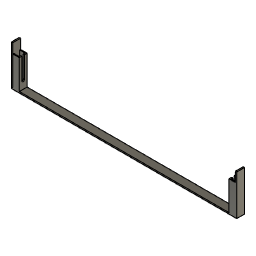
motor_base1 v1 (Autodesk Fusion 360 design; units mm, degrees)
Autodesk Fusion 360 part; units mm, degrees
sketch "Sketch1" plane through (0, 0, 0) normal (0, 0, 1) x (1, 0, 0)
  line L0 (-173, 6) -> (173, 6)
  line L1 (173, 6) -> (173, -6)
  line L2 (173, -6) -> (-173, -6)
  line L3 (-173, -6) -> (-173, 6)
  dimension "d1" = 346
  dimension "d2" = 12
  constraint horizontal L0
  constraint perpendicular L0 L1
  constraint parallel L0 L2
  constraint parallel L1 L3
  measures "d1" distance of L0.start L0.end
  measures "d2" distance of L0.end L1.end
extrude "Extrude1" add sketch "Sketch1" along normal blind 2
sketch "Sketch2" plane through (0, 0, 2) normal (0, 0, 1) x (-1, 0, 0)
  line L0 (173, 6) -> (-173, 6)
  line L1 (-173, 6) -> (-173, -6)
  line L2 (-173, -6) -> (173, -6)
  line L3 (173, -6) -> (173, 6)
  line L4 (-171, 6) -> (-171, -6)
  line L5 (-171, 6) -> (-173, 6)
  line L6 (-173, -6) -> (-171, -6)
  line L7 (171, 6) -> (171, -6)
  line L8 (171, 6) -> (173, 6)
  line L9 (173, -6) -> (171, -6)
  dimension "d9" = 2
  dimension "d10" = 2
  constraint coincident L0 L4.start
  constraint perpendicular L0 L4
  constraint coincident L0.end L1.start
  constraint coincident L1.end L2.start
  constraint coincident L0 L7.start
  constraint coincident L2 L7.end
  constraint perpendicular L2 L7
  constraint coincident L0.start L3.end
  constraint coincident L2.end L3.start
  measures "d9" distance of L1 L4
  measures "d10" distance of L3 L7
extrude "Extrude2" add sketch "Sketch2" along normal blind 60 contours L0 L2 L3 L7 L8 L9 | L0 L1 L2 L4 L5 L6
sketch "Sketch3" plane through (171, 0, 0) normal (-1, 0, 0) x (0, -1, 0)
  line L0 (-6, 2) -> (6, 2)
  line L1 (6, 2) -> (6, 62)
  line L2 (6, 62) -> (-6, 62)
  line L3 (-6, 62) -> (-6, 2)
  line L4 (-6, 62) -> (-6, 47)
  line L5 (-6, 47) -> (6, 47)
  line L6 (6, 47) -> (6, 0)
  line L7 (6, 0) -> (-6, 0)
  line L8 (-6, 0) -> (-6, 47)
  dimension "d13" = 15
  constraint coincident L2.end L3.start
  constraint perpendicular L2 L4
  constraint coincident L1 L5.end
  constraint perpendicular L1 L5
  constraint perpendicular L0 L6
  constraint perpendicular L3 L7
  constraint perpendicular L5 L8
  measures "d13" distance of L2.end L4.end
extrude "Extrude3" add sketch "Sketch3" along normal blind 10 contours L0 L1 L3 L5 L6 L8
sketch "Sketch4" plane through (0, 0, 47) normal (0, 0, 1) x (-1, 0, 0)
  line L0 (-171, 6) -> (-171, -6)
  line L1 (-171, -6) -> (-161, -6)
  line L2 (-161, -6) -> (-161, 6)
  line L3 (-161, 6) -> (-171, 6)
  line L4 (-171, 4.5) -> (-170, 4.5)
  line L5 (-170, 4.5) -> (-163, 4.5)
  line L6 (-163, 4.5) -> (-163, -4.5)
  line L7 (-163, -4.5) -> (-171, -4.5)
  line L8 (-171, 4.5) -> (-171, 3.6158)
  dimension "d16" = 1.5
  dimension "d17" = 1.5
  dimension "d18" = 8
  constraint coincident L0 L4.start
  constraint perpendicular L0 L4
  constraint perpendicular L0 L5
  constraint perpendicular L4 L6
  constraint coincident L0 L7.end
  constraint perpendicular L0 L7
  constraint coincident L0 L8.end
  measures "d16" distance of L3 L5
  measures "d17" distance of L1 L7
  measures "d18" distance of L6.end L7.end
extrude "Extrude4" cut sketch "Sketch4" against normal blind 43 contours L0 L4 L5 L6 L7 L8
sketch "Sketch5" plane through (161, 0, 0) normal (-1, 0, 0) x (0, -1, 0)
  line L0 (-6, 47) -> (-6, 2)
  line L1 (-6, 2) -> (6, 2)
  line L2 (6, 2) -> (6, 47)
  line L3 (6, 47) -> (-6, 47)
  line L4 (-6, 47) -> (6, 47)
  line L5 (0, 47) -> (-2, 47)
  line L6 (3, 12) -> (3, 13.1676)
  line L7 (-2, 47) -> (-2, 14)
  line L8 (2, 14) -> (2, 47)
  line L9 (2, 47) -> (-2, 47)
  arc A0 (0, 12) -> (2, 14) centre (0, 14) ccw
  arc A1 (-2, 14) -> (0, 12) centre (0, 14) ccw
  point P0 (-2, 12)
  point P1 (3.9688, 12.6113)
  point P2 (-2, 12)
  point P3 (2, 12)
  dimension "d21" = 2
  dimension "d30" = 35
  dimension "d31" = 4
  dimension "d32" = 35
  dimension "d33" = 2
  dimension "d34" = 2
  constraint coincident L0.start L3.end
  constraint coincident L2.end L3.start
  constraint midpoint L4 L5.start
  constraint perpendicular L0 L5
  constraint perpendicular L5 L7
  constraint coincident P3 L8
  constraint tangent L8 A0
  constraint coincident P2 L7
  constraint tangent L7 A1
  constraint coincident A0.start A1.end
  measures "d21" distance of L5.start L5.end
  measures "d30" distance of L5.end P2
  measures "d31" distance of P2 P3
  measures "d32" distance of P3 L8.end
  measures "d33" radius of A0
  measures "d34" radius of A1
extrude "Extrude5" cut sketch "Sketch5" against normal blind 2 contours L3 L4 L5 L7 L8 L9 A0 A1
sketch "Sketch6" plane through (-171, 0, 0) normal (1, 0, 0) x (0, 1, 0)
  line L0 (-6, 2) -> (6, 2)
  line L1 (6, 2) -> (6, 62)
  line L2 (6, 62) -> (-6, 62)
  line L3 (-6, 62) -> (-6, 2)
  line L4 (-6, 62) -> (-6, 47)
  line L5 (-6, 47) -> (6, 47)
  line L6 (-6, 47) -> (-6, 0)
  line L7 (-6, 0) -> (6, 0)
  line L8 (6, 0) -> (6, 47)
  dimension "d37" = 15
  constraint coincident L2.end L3.start
  constraint perpendicular L2 L4
  constraint coincident L1 L5.end
  constraint perpendicular L1 L5
  constraint perpendicular L0 L6
  constraint perpendicular L1 L7
  constraint perpendicular L5 L8
  measures "d37" distance of L2.end L4.end
extrude "Extrude6" add sketch "Sketch6" along normal blind 10 contours L0 L1 L3 L5 L6 L8
sketch "Sketch7" plane through (0, 0, 47) normal (0, 0, 1) x (-1, 0, 0)
  line L0 (171, -6) -> (171, 6)
  line L1 (171, 6) -> (161, 6)
  line L2 (161, 6) -> (161, -6)
  line L3 (161, -6) -> (171, -6)
  line L4 (171, 4.5) -> (163, 4.5)
  line L5 (163, 4.5) -> (163, -4.5)
  line L6 (163, -4.5) -> (171, -4.5)
  dimension "d40" = 1.5
  dimension "d41" = 1.5
  dimension "d42" = 2
  constraint coincident L0 L4.start
  constraint perpendicular L0 L4
  constraint perpendicular L4 L5
  constraint coincident L0 L6.end
  constraint perpendicular L0 L6
  measures "d40" distance of L3 L6
  measures "d41" distance of L1 L4
  measures "d42" distance of L2 L5
extrude "Extrude7" cut sketch "Sketch7" against normal blind 43 contours L0 L4 L5 L6
sketch "Sketch8" plane through (-161, 0, 0) normal (1, 0, 0) x (0, 1, 0)
  line L0 (-6, 47) -> (-6, 2)
  line L1 (-6, 2) -> (6, 2)
  line L2 (6, 2) -> (6, 47)
  line L3 (6, 47) -> (-6, 47)
  line L4 (6, 47) -> (-6, 47)
  line L5 (0, 47) -> (-2, 47)
  line L6 (-2, 47) -> (-2, 14)
  line L7 (2, 14) -> (2, 47)
  line L8 (2, 47) -> (-2, 47)
  arc A0 (-2, 14) -> (0, 12) centre (0, 14) ccw
  arc A1 (0, 12) -> (2, 14) centre (0, 14) ccw
  point P0 (-2, 12)
  point P1 (2, 12)
  dimension "d45" = 2
  dimension "d46" = 35
  dimension "d47" = 4
  dimension "d48" = 35
  dimension "d49" = 2
  dimension "d50" = 2
  constraint coincident L2.end L3.start
  constraint coincident L0.start L3.end
  constraint midpoint L4 L5.start
  constraint perpendicular L2 L5
  constraint perpendicular L4 L6
  constraint coincident P0 L6
  constraint tangent L6 A0
  constraint coincident P1 L7
  constraint tangent L7 A1
  constraint coincident A0.end A1.start
  measures "d45" distance of L5.start L5.end
  measures "d46" distance of L5.end P0
  measures "d47" distance of P0 P1
  measures "d48" distance of P1 L7.end
  measures "d49" radius of A0
  measures "d50" radius of A1
extrude "Extrude8" cut sketch "Sketch8" against normal blind 2 contours L3 L4 L5 L6 L7 L8 A0 A1
